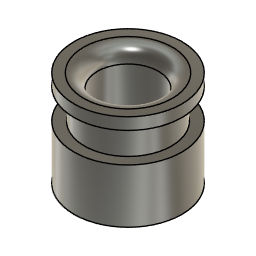
pingpong_motor_attachment_1 v2 (Autodesk Fusion 360 design; units mm, degrees)
Autodesk Fusion 360 part; units mm, degrees
sketch "Sketch1" plane through (0, 0, 0) normal (0, 0, 1) x (1, 0, 0)
  circle A0 centre (0, 0) radius 12.5
  circle A1 centre (0, 0) radius 8.75
  circle A2 centre (0, 0) radius 15.5
  dimension "d1" = 17.5
  dimension "d2" = 25
  dimension "d3" = 3
  constraint coincident A0.centre A1.centre
  measures "d1" diameter of A1
  measures "d2" diameter of A0
extrude "Extrude1" add sketch "Sketch1" along normal blind 20 contours A0 | A2
fillet "Fillet1" radius 4 2 edges at (-8.1579, 3.1641, 20) (-8.1579, 3.1641, 0)
extrude "Extrude2" cut sketch "Sketch1" along normal blind 8.6 from surface at 8 contours A2
move_face "OffsetFaces1" offset 7.5 1 faces at (14.4782, -1.4035, 0)
